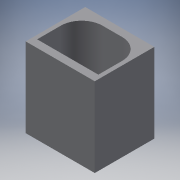
# Autodesk Inventor part: thermostatBath
Saved by Autodesk Inventor 2017 (Build 210142000, 142)
## iProperties
Created: 2016-11-02
Part Number: thermostatBath
Material: Generic
Document SubType Name: Modeling
Designer: Camilo
Density: 1 g/cm^3
Appearance: Default
Author: Camilo
Autodesk Inventor part; units mm, degrees
ref_plane "YZ Plane" through (0, 0, 0) normal (1, 0, 0) x (0, 1, 0)
ref_plane "XZ Plane" through (0, 0, 0) normal (0, 1, 0) x (-1, 0, 0)
ref_plane "XY Plane" through (0, 0, 0) normal (0, 0, 1) x (1, 0, 0)
sketch "Sketch2" plane through (0, 0, 0) normal (0, 0, 1) x (1, 0, 0)
  line L0 (87, 75) -> (-87, 75)
  line L1 (-87, 75) -> (-87, -75)
  line L2 (-87, -75) -> (87, -75)
  line L3 (87, -75) -> (87, 75)
  line L4 (87, 75) -> (-87, -75) construction
  line L5 (-87, 75) -> (87, -75) construction
  point P0 (0, 0)
  dimension "d3" = 174
  dimension "d4" = 150
  constraints: 12 end point, 2 midpoint, 2 parallel, 1 horizontal, 1 perpendicular
  measures "d3" distance of L0.start L0.end
  measures "d4" distance of L1.end L0.end
sketch "Sketch1" plane through (0, 0, 0) normal (0, 0, 1) x (1, 0, 0)
  line L0 (77, 56) -> (-77, 56)
  line L1 (-77, 56) -> (-77, -56)
  line L2 (-77, -56) -> (77, -56)
  line L3 (77, -56) -> (77, 56)
  line L4 (77, 56) -> (-77, -56) construction
  line L5 (-77, 56) -> (77, -56) construction
  arc A0 (77, 3.5816) -> (24.5816, 56) centre (24.5816, 3.5816) ccw
  line L6 (-77, -56) -> (59.13, 43.0036) construction
  arc A1 (-24.5816, 56) -> (-77, 3.5816) centre (-24.5816, 3.5816) ccw
  point P0 (0, 0)
  dimension "d0" = 154
  dimension "d1" = 112
  dimension "d2" = 136.13
  constraints: 14 end point, 5 point on circle, 5 point on line, 4 tangent, 2 centre point, 2 midpoint, 2 parallel, 1 equal radius, 1 horizontal, 1 perpendicular
  measures "d0" distance of L0.start L0.end
  measures "d1" distance of L1.end L0.end
  measures "d2" horizontal distance of L1.end L6.end
extrude "Extrusion1" add sketch "Sketch2" against normal blind 200
extrude "Extrusion2" cut sketch "Sketch1" against normal blind 150 contours A0 L3 L2 L1 A1 L0
body "Solid1"
